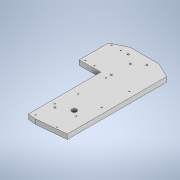
# Autodesk Inventor part: montageplaatje
Saved by Autodesk Inventor 2021 (Build 250183000, 183)
## iProperties
Created: 2022-11-09
Part Number: montageplaatje
Material: Generic
Document SubType Name: Modeling
Designer: marti
Density: 1 g/cm^3
Appearance: Default
Author: marti
Autodesk Inventor part; units mm, degrees
ref_plane "YZ Plane" through (0, 0, 0) normal (1, 0, 0) x (0, 1, 0)
ref_plane "XZ Plane" through (0, 0, 0) normal (0, 1, 0) x (-1, 0, 0)
ref_plane "XY Plane" through (0, 0, 0) normal (0, 0, 1) x (1, 0, 0)
sketch "Sketch1" plane through (0, 0, 0) normal (0, 1, 0) x (-1, 0, 0)
  line L0 (19.5, -173) -> (0, -173) construction
  line L1 (0, -173) -> (-19.5, -173) construction
  line L2 (61, -173) -> (61, 35)
  line L3 (0, 0) -> (0, -173) construction
  line L4 (0, -188) -> (30, -188)
  line L5 (61, -173) -> (30, -188)
  line L6 (61, 35) -> (0, 41)
  line L7 (-61, -173) -> (-61, 35)
  line L8 (0, -188) -> (-30, -188)
  line L9 (-61, -173) -> (-30, -188)
  line L10 (-61, 35) -> (0, 41)
  point P0 (0, -118)
  point P1 (0, -158)
  dimension "d0" = 118
  dimension "d1" = 40
  dimension "d2" = 19.5
  dimension "d3" = 15
  dimension "d4" = 61
  dimension "d6" = 15
  dimension "d7" = 35
  dimension "d8" = 41
  dimension "d11" = 30
  constraints: 22 end point, 4 vertical alignment, 3 symmetric about line, 2 collinear, 2 horizontal, 2 vertical, 1 coincident, 1 horizontal alignment
  measures "d0" distance of point (0, 0) point (0, -118)
  measures "d1" distance of point (0, -118) point (0, -158)
  measures "d2" horizontal distance of point (0, -158) L0.start
  measures "d3" vertical distance of point (0, -158) L0.start
  measures "d4" distance between parallel lines of L3 L2
  measures "d6" distance from line of L0.start L4
  measures "d7" vertical distance of L2.end L3.start
  measures "d8" distance of L3.start L6.end
  measures "d11" horizontal distance of L0.end L4.end
extrude "uitlijn plaatje" add sketch "Sketch1" along normal blind 10
hole "Hole1" at (-19.5, 0, -173) at (19.5, 0, -173) at (0, 0, 0) at (0, 0, -118) at (0, 0, -158) direction (0, 1, 0) diameter 3.4 end through all clearance for "Hex Head Cap Screw ISO 24017" size "M3" standard "ISO"
sketch "batterij uitsnijding" plane through (0, 10, 0) normal (0, 1, 0) x (1, 0, 0)
  line L0 (-61, -35) -> (0, -41) projected
  line L1 (-16, -39.4262) -> (-16, 112)
  line L2 (-16, 112) -> (-61, 112)
  line L3 (-61, 173) -> (-61, -35) projected
  point P0 (0, 0)
  dimension "d21" = 45
  dimension "d22" = 112
  constraints: 4 end point, 1 perpendicular, 1 point on line, 1 vertical
  measures "d21" distance between parallel lines of L3 L1
  measures "d22" distance from line of point (0, 0) L2
extrude "Extrusion2" cut sketch "batterij uitsnijding" against normal blind 10
sketch "Sketch3" plane through (0, 10, 0) normal (0, 1, 0) x (1, 0, 0)
  circle A0 centre (25.75, 14.75) radius 5
  point P0 (0, 0)
  dimension "d26" = 14.75
  dimension "d27" = 25.75
  dimension "d28" = 10
  constraints: 1 centre point
  measures "d26" vertical distance of A0.centre point (0, 0)
  measures "d27" horizontal distance of A0.centre point (0, 0)
  measures "d28" diameter of A0
extrude "Extrusion3" cut sketch "Sketch3" against normal blind 10
sketch "Sketch4" plane through (0, 10, 0) normal (0, 1, 0) x (1, 0, 0)
  line L0 (56.6557, 130.4025) -> (-9.4519, 130.4025)
  line L1 (-9.4519, 130.4025) -> (-9.4519, 45.4025)
  line L2 (-9.4519, 45.4025) -> (56.6557, 45.4025)
  line L3 (56.6557, 45.4025) -> (56.6557, 130.4025)
  point P0 (0, 0)
  point P1 (-6.8294, -33.3939)
  point P2 (-6.8294, 6.6061)
  point P3 (38.1706, -33.3939)
  point P4 (38.1706, 6.6061)
  point P5 (-34.5164, 117.3451)
  point P6 (-53.5164, 117.3451)
  point P7 (-34.5164, 172.3451)
  point P8 (-53.5164, 172.3451)
  point P9 (0, 48.9025)
  point P10 (49, 48.9025)
  point P11 (49, 106.9025)
  point P12 (0, 106.9025)
  dimension "d31" = 40
  dimension "d32" = 45
  dimension "d33" = 19
  dimension "d34" = 55
  dimension "d35" = 58
  dimension "d36" = 49
  dimension "d37" = 55
  dimension "d38" = 19
  dimension "d39" = 85
  dimension "d40" = 3.5
  constraints: 8 end point, 5 horizontal alignment, 5 vertical alignment, 2 parallel, 1 horizontal, 1 perpendicular
  measures "d31" distance of point (-6.829, 6.606) point (-6.829, -33.394)
  measures "d32" distance of point (38.171, -33.394) point (-6.829, -33.394)
  measures "d33" distance of point (-53.516, 117.345) point (-34.516, 117.345)
  measures "d34" distance of point (-34.516, 117.345) point (-34.516, 172.345)
  measures "d35" distance of point (0, 106.902) point (0, 48.902)
  measures "d36" distance of point (49, 48.902) point (0, 48.902)
  measures "d37" distance of point (-53.516, 117.345) point (-53.516, 172.345)
  measures "d38" distance of point (-34.516, 172.345) point (-53.516, 172.345)
  measures "d39" distance of L0.end L1.end
  measures "d40" distance from line of L2 point (0, 48.902)
hole "Hole2" at (-6.8294, 10, 33.3939) at (-6.8294, 10, -6.6061) at (38.1706, 10, 33.3939) at (38.1706, 10, -6.6061) at (-34.5164, 10, -117.3451) at (-53.5164, 10, -117.3451) at (-34.5164, 10, -172.3451) at (-53.5164, 10, -172.3451) at (0, 10, -48.9025) at (49, 10, -48.9025) at (49, 10, -106.9025) at (0, 10, -106.9025) direction (0, -1, 0) diameter 2.2 end through all
body "Solid1"
